Autodesk Inventor part; units mm, degrees
(part 2 of 2)
  line L705 (120.1659, 1.1) -> (121.7367, 1.1) construction
  line L706 (119.8111, 0.125) -> (120.5299, 2.1)
  line L707 (121.3727, 2.1) -> (122.0916, 0.125)
  line L708 (120.9513, 2.1) -> (120.9513, 0) construction
  line L709 (120.5299, 2.1) -> (121.3727, 2.1)
  line L710 (119.6325, 0) -> (122.2701, 0) construction
  arc A175 (119.6325, 0) -> (119.8111, 0.125) centre (119.6325, 0.19) ccw
  line L711 (119.3805, 0) -> (119.6325, 0)
  line L712 (125.4117, 0) -> (125.6637, 0)
  arc A176 (125.2332, 0.125) -> (125.4117, 0) centre (125.4117, 0.19) ccw
  line L713 (123.3075, 1.1) -> (124.8783, 1.1) construction
  line L714 (122.9526, 0.125) -> (123.6715, 2.1)
  line L715 (124.5143, 2.1) -> (125.2332, 0.125)
  line L716 (124.0929, 2.1) -> (124.0929, 0) construction
  line L717 (123.6715, 2.1) -> (124.5143, 2.1)
  line L718 (122.7741, 0) -> (125.4117, 0) construction
  arc A177 (122.7741, 0) -> (122.9526, 0.125) centre (122.7741, 0.19) ccw
  line L719 (122.5221, 0) -> (122.7741, 0)
  line L720 (128.5533, 0) -> (128.8053, 0)
  arc A178 (128.3748, 0.125) -> (128.5533, 0) centre (128.5533, 0.19) ccw
  line L721 (126.4491, 1.1) -> (128.0199, 1.1) construction
  line L722 (126.0942, 0.125) -> (126.8131, 2.1)
  line L723 (127.6559, 2.1) -> (128.3748, 0.125)
  line L724 (127.2345, 2.1) -> (127.2345, 0) construction
  line L725 (126.8131, 2.1) -> (127.6559, 2.1)
  line L726 (125.9157, 0) -> (128.5533, 0) construction
  arc A179 (125.9157, 0) -> (126.0942, 0.125) centre (125.9157, 0.19) ccw
  line L727 (125.6637, 0) -> (125.9157, 0)
  line L728 (131.6949, 0) -> (131.9469, 0)
  arc A180 (131.5164, 0.125) -> (131.6949, 0) centre (131.6949, 0.19) ccw
  line L729 (129.5907, 1.1) -> (131.1615, 1.1) construction
  line L730 (129.2358, 0.125) -> (129.9547, 2.1)
  line L731 (130.7975, 2.1) -> (131.5164, 0.125)
  line L732 (130.3761, 2.1) -> (130.3761, 0) construction
  line L733 (129.9547, 2.1) -> (130.7975, 2.1)
  line L734 (129.0573, 0) -> (131.6949, 0) construction
  arc A181 (129.0573, 0) -> (129.2358, 0.125) centre (129.0573, 0.19) ccw
  line L735 (128.8053, 0) -> (129.0573, 0)
  line L736 (134.8365, 0) -> (135.0885, 0)
  arc A182 (134.658, 0.125) -> (134.8365, 0) centre (134.8365, 0.19) ccw
  line L737 (132.7323, 1.1) -> (134.3031, 1.1) construction
  line L738 (132.3774, 0.125) -> (133.0963, 2.1)
  line L739 (133.9391, 2.1) -> (134.658, 0.125)
  line L740 (133.5177, 2.1) -> (133.5177, 0) construction
  line L741 (133.0963, 2.1) -> (133.9391, 2.1)
  line L742 (132.1989, 0) -> (134.8365, 0) construction
  arc A183 (132.1989, 0) -> (132.3774, 0.125) centre (132.1989, 0.19) ccw
  line L743 (131.9469, 0) -> (132.1989, 0)
  line L744 (137.9781, 0) -> (138.2301, 0)
  arc A184 (137.7995, 0.125) -> (137.9781, 0) centre (137.9781, 0.19) ccw
  line L745 (135.8739, 1.1) -> (137.4447, 1.1) construction
  line L746 (135.519, 0.125) -> (136.2379, 2.1)
  line L747 (137.0807, 2.1) -> (137.7995, 0.125)
  line L748 (136.6593, 2.1) -> (136.6593, 0) construction
  line L749 (136.2379, 2.1) -> (137.0807, 2.1)
  line L750 (135.3405, 0) -> (137.9781, 0) construction
  arc A185 (135.3405, 0) -> (135.519, 0.125) centre (135.3405, 0.19) ccw
  line L751 (135.0885, 0) -> (135.3405, 0)
  line L752 (141.1197, 0) -> (141.3717, 0)
  arc A186 (140.9411, 0.125) -> (141.1197, 0) centre (141.1197, 0.19) ccw
  line L753 (139.0155, 1.1) -> (140.5863, 1.1) construction
  line L754 (138.6606, 0.125) -> (139.3794, 2.1)
  line L755 (140.2223, 2.1) -> (140.9411, 0.125)
  line L756 (139.8009, 2.1) -> (139.8009, 0) construction
  line L757 (139.3794, 2.1) -> (140.2223, 2.1)
  line L758 (138.4821, 0) -> (141.1197, 0) construction
  arc A187 (138.4821, 0) -> (138.6606, 0.125) centre (138.4821, 0.19) ccw
  line L759 (138.2301, 0) -> (138.4821, 0)
  line L760 (144.2613, 0) -> (144.5133, 0)
  arc A188 (144.0827, 0.125) -> (144.2613, 0) centre (144.2613, 0.19) ccw
  line L761 (142.1571, 1.1) -> (143.7279, 1.1) construction
  line L762 (141.8022, 0.125) -> (142.521, 2.1)
  line L763 (143.3639, 2.1) -> (144.0827, 0.125)
  line L764 (142.9425, 2.1) -> (142.9425, 0) construction
  line L765 (142.521, 2.1) -> (143.3639, 2.1)
  line L766 (141.6237, 0) -> (144.2613, 0) construction
  arc A189 (141.6237, 0) -> (141.8022, 0.125) centre (141.6237, 0.19) ccw
  line L767 (141.3717, 0) -> (141.6237, 0)
  line L768 (147.4029, 0) -> (147.6549, 0)
  arc A190 (147.2243, 0.125) -> (147.4029, 0) centre (147.4029, 0.19) ccw
  line L769 (145.2987, 1.1) -> (146.8695, 1.1) construction
  line L770 (144.9438, 0.125) -> (145.6626, 2.1)
  line L771 (146.5055, 2.1) -> (147.2243, 0.125)
  line L772 (146.0841, 2.1) -> (146.0841, 0) construction
  line L773 (145.6626, 2.1) -> (146.5055, 2.1)
  line L774 (144.7653, 0) -> (147.4029, 0) construction
  arc A191 (144.7653, 0) -> (144.9438, 0.125) centre (144.7653, 0.19) ccw
  line L775 (144.5133, 0) -> (144.7653, 0)
  line L776 (150.5445, 0) -> (150.7964, 0)
  arc A192 (150.3659, 0.125) -> (150.5445, 0) centre (150.5445, 0.19) ccw
  line L777 (148.4403, 1.1) -> (150.011, 1.1) construction
  line L778 (148.0854, 0.125) -> (148.8042, 2.1)
  line L779 (149.6471, 2.1) -> (150.3659, 0.125)
  line L780 (149.2257, 2.1) -> (149.2257, 0) construction
  line L781 (148.8042, 2.1) -> (149.6471, 2.1)
  line L782 (147.9068, 0) -> (150.5445, 0) construction
  arc A193 (147.9068, 0) -> (148.0854, 0.125) centre (147.9068, 0.19) ccw
  line L783 (147.6549, 0) -> (147.9068, 0)
  line L784 (153.686, 0) -> (153.938, 0)
  arc A194 (153.5075, 0.125) -> (153.686, 0) centre (153.686, 0.19) ccw
  line L785 (151.5818, 1.1) -> (153.1526, 1.1) construction
  line L786 (151.227, 0.125) -> (151.9458, 2.1)
  line L787 (152.7887, 2.1) -> (153.5075, 0.125)
  line L788 (152.3672, 2.1) -> (152.3672, 0) construction
  line L789 (151.9458, 2.1) -> (152.7887, 2.1)
  line L790 (151.0484, 0) -> (153.686, 0) construction
  arc A195 (151.0484, 0) -> (151.227, 0.125) centre (151.0484, 0.19) ccw
  line L791 (150.7964, 0) -> (151.0484, 0)
  point P0 (0, 0)
  point P1 (-18.8496, 0)
  point P2 (-15.708, 0)
  point P3 (-12.5664, 0)
  point P4 (-3.1416, 0)
  point P5 (120.9513, 0)
  point P6 (149.2257, 0)
  point P7 (152.3672, 0)
  dimension "d52" = 40
  dimension "d53" = 1
  dimension "d54" = 1.5708
  dimension "d55" = 1.5708
  dimension "d56" = 0.19
  dimension "d57" = 1.1
  dimension "d58" = 1.5708
  dimension "d61" = 3.1416
  constraints: 1578 end point, 492 point on line, 392 point on circle, 196 centre point, 5 horizontal, 4 tangent, 3 midpoint, 3 parallel, 3 vertical, 1 coincident, 1 collinear, 1 equal length, 1 perpendicular, 2426 other
  measures "d52" angle of L6 L4
  measures "d53" distance between parallel lines of L5 L10
  measures "d54" distance between parallel lines of L0 L8
  measures "d55" distance from line of L8 L7.end
  measures "d56" radius of A1
  measures "d57" distance between parallel lines of L10 L1
  measures "d58" distance of L10.end L10.start
  measures "d61" distance of L8.end L15.end
extrude "Zahnprofil" cut sketch "Skizze5" against normal through all
sketch "Skizze4" plane through (6, -5.9, 153.938) normal (1, 0, 0) x (0, 0, -1)
  line L0 (159.798, 12.6836) -> (48.4645, 12.6836)
  line L1 (48.4645, 12.6836) -> (48.4645, -7.7347)
  line L2 (48.4645, -7.7347) -> (159.798, -7.7347)
  line L3 (159.798, -7.7347) -> (159.798, 12.6836)
  point P0 (153.938, 5.9)
  constraints: 8 end point, 2 parallel, 1 horizontal, 1 perpendicular
extrude "Extrusion4" [suppressed]
ref_plane "Arbeitsebene1" through (3, 0, 0) normal (1, 0, 0) x (0, 0, -1)
ref_plane "Arbeitsebene6" through (6, 0, 34.5575) normal (0, 1, 0) x (1, 0, 0)
ref_plane "Arbeitsebene3" through (6, 1.1, -115.0896) normal (0, 1, 0) x (-1, 0, 0)
ref_plane "Arbeitsebene2" through (6, 2.1, -115.0896) normal (0, 1, 0) x (-1, 0, 0)
ref_plane "Arbeitsebene7" through (0, -5.9, 0) normal (0, 0, 1) x (1, 0, 0)
sketch "Skizze13" plane through (6, -5.9, 153.938) normal (0, 0, -1) x (-1, 0, 0)
  line L0 (0, 5.9) -> (0, 0) projected
  line L1 (6, 0) -> (0, 0) projected
  line L2 (6, 5.9) -> (6, 0) projected
  line L3 (6, 5.9) -> (0, 5.9) projected
  point P0 (6, 5.9)
extrude "Extrusion12" add sketch "Skizze13" against normal blind 2.6239
sketch "Skizze14" plane through (0, -5.9, -153.938) normal (0, -1, 0) x (1, 0, 0)
  line L0 (0, 0) -> (6, 0) construction
  line L1 (6, 0) -> (6, 310.5) construction
  line L2 (0, 310.5) -> (6, 310.5) construction
  line L3 (0, 0) -> (0, 310.5) construction
  line L4 (3, 372.6) -> (3, -62.1) construction
  point P0 (0, 153.938)
  point P1 (3, 25.1327)
  point P2 (3, 76.0265)
  point P3 (3, 126.9203)
  point P4 (3, 177.8141)
  point P5 (3, 228.7079)
  point P6 (3, 279.6017)
  dimension "d97" = 25.1327
  dimension "d98" = 310.5
  dimension "d101" = 50.8938
  constraints: 1 point on line, 1 vertical, 5 other
  measures "d97" distance from line of L0 point (3, 25.133)
  measures "d98" distance between parallel lines of L2 L0
  measures "d101" distance of point (3, 25.133) point (3, 76.027)
hole "Bohrung2" at (3, -5.9, -128.8053) at (3, -5.9, -77.9115) at (3, -5.9, -27.0177) at (3, -5.9, 23.8761) at (3, -5.9, 74.7699) at (3, -5.9, 125.6637) direction (0, 1, 0) diameter 2.459 depth 5.2 thread size "M3x0.5" class "6H" standard "ISO Metric profile"
split body "Trennen3" result two bodies by plane through (0, -5.9, 0) normal (0, 0, 1) first body at (0.5, -3.9333, 93.112)
sketch "Skizze12" plane through (0, 0, 0) normal (0, 0, -1) x (-1, 0, 0)
  line L0 (0, -2.95) -> (-6, -2.95) construction
  line L1 (-3, -5.9) -> (-3, -2.95) construction
  circle A0 centre (-3, -2.95) radius 1.5
  line L2 (-6, 0) -> (-6, -5.9) construction
  line L3 (-6, -5.9) -> (0, -5.9) construction
  line L4 (0, -5.9) -> (0, 0) construction
  point P0 (-6, 2.1)
  point P1 (0, 2.1)
  dimension "d91" = 3
  dimension "d96" = 2.95
  constraints: 4 end point, 3 midpoint, 1 centre point, 1 coincident, 1 vertical
  measures "d91" diameter of A0
  measures "d96" distance between parallel lines of L0 L3
extrude "Extrusion11" cut sketch "Skizze12" along normal mid plane 25 bodies 2 3
sketch "Sketch15" plane through (6, -5.9, 156.562) normal (0, 0, 1) x (1, 0, 0)
  circle A0 centre (-3, 2.95) radius 0.5
  line L0 (-6, 5.9) -> (-6, 0) projected
  line L1 (-6, 2.95) -> (0, 2.95) construction
  line L2 (0, 0) -> (0, 5.9) projected
  line L3 (-3, 19.08) -> (-3, -3.18) construction
  dimension "d114" = 1
  constraints: 3 midpoint, 2 end point, 1 centre point, 1 point on line
  measures "d114" diameter of A0
extrude "Bottom_Mark" cut sketch "Sketch15" against normal blind 1 bodies 2
equation "\"Kopfspiel\" = 0.1"
equation "\"Modul\" = 1"
equation "\"Fussrundung\" = 0.38"
equation "\"Teilung\" = 3.14159"
